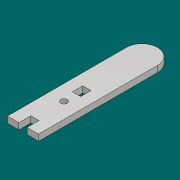
# Autodesk Inventor part: gpu_support
Saved by Autodesk Inventor 2018.2 (Build 222227000, 227)
## iProperties
Created: 2020-08-09
Part Number: gpu_support
Material: アルミニウム 6061
Document SubType Name: Modeling
Designer: gisen
Density: 2.7 g/cm^3
Appearance: アルミニウム - フラット
Author: gisen
Autodesk Inventor part; units mm, degrees
ref_plane "YZ Plane" through (0, 0, 0) normal (1, 0, 0) x (0, 1, 0)
ref_plane "XZ Plane" through (0, 0, 0) normal (0, 1, 0) x (-1, 0, 0)
ref_plane "XY Plane" through (0, 0, 0) normal (0, 0, 1) x (1, 0, 0)
sketch "スケッチ1" plane through (0, 0, 0) normal (0, 0, 1) x (1, 0, 0)
  line L0 (0, 0) -> (5.5, 0)
  line L1 (5.5, 0) -> (5.5, 6)
  line L2 (5.5, 6) -> (9.5, 6)
  line L3 (9.5, 6) -> (9.5, 0)
  line L4 (9.5, 0) -> (15, 0)
  line L5 (15, 0) -> (15, 57.5)
  arc A0 (15, 57.5) -> (0, 57.5) centre (7.5, 57.5) ccw
  line L6 (0, 0) -> (0, 57.5)
  line L7 (15, 57.5) -> (0, 57.5) construction
  line L8 (7.5, 6) -> (7.5, 20) construction
  circle A1 centre (7.5, 20) radius 1.6
  line L9 (5.5, 26) -> (9.5, 26)
  line L10 (9.5, 26) -> (9.5, 31)
  line L11 (9.5, 31) -> (5.5, 31)
  line L12 (5.5, 31) -> (5.5, 26)
  line L13 (7.5, 57.5) -> (7.5, 65) construction
  dimension "d0" = 4
  dimension "d1" = 6
  dimension "d2" = 15
  dimension "d3" = 20
  dimension "d4" = 3.2
  dimension "d5" = 26
  dimension "d6" = 5
  dimension "d7" = 65
  constraints: 28 end point, 5 perpendicular, 4 point on line, 3 horizontal, 3 point on circle, 2 centre point, 2 coincident, 2 midpoint, 2 parallel, 1 collinear, 1 tangent, 1 vertical
  measures "d0" distance of L1.end L2.end
  measures "d1" distance of L2.end L3.end
  measures "d2" distance between parallel lines of L5 L6
  measures "d3" distance from line of L4 L8.end
  measures "d4" diameter of A1
  measures "d5" distance between parallel lines of L4 L9
  measures "d6" distance of L9.end L10.end
  measures "d7" vertical distance of L0.start L13.end
extrude "押し出し1" add sketch "スケッチ1" along normal blind 3
sketch "スケッチ2" plane through (0, 0, 3) normal (0, 0, 1) x (1, 0, 0)
  point P0 (0, 0)
sketch "スケッチ3" plane through (0, 0, 3) normal (0, 0, 1) x (1, 0, 0)
  line L0 (0, 0) -> (5.5, 0) projected
  line L1 (0, 0) -> (5.5, 0)
  line L2 (5.5, 0) -> (5.5, 0.25)
  line L3 (5.5, 0.25) -> (0, 0.25)
  line L4 (0, 0.25) -> (0, 0)
  line L5 (9.5, 0) -> (15, 0) projected
  line L6 (9.5, 6) -> (9.5, 0) projected
  line L7 (15, 0) -> (9.5, 0)
  line L8 (9.5, 0) -> (9.5, 0.25)
  line L9 (9.5, 0.25) -> (15, 0.25)
  line L10 (15, 0.25) -> (15, 0)
  line L11 (5.5, 0) -> (5.5, 6) projected
  dimension "d10" = 0.25
  dimension "d11" = 0.25
  constraints: 16 end point, 4 parallel, 2 horizontal, 2 perpendicular, 2 point on line
  measures "d10" distance between parallel lines of L0 L3
  measures "d11" distance between parallel lines of L5 L9
extrude "押し出し2" cut sketch "スケッチ3" against normal through all
equation "\"d11\" = d10"
